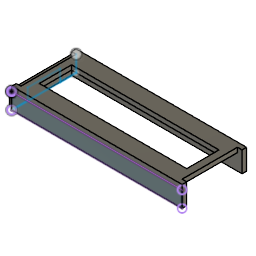
LCD Schutz (Autodesk Fusion 360 design; units mm, degrees)
part number: 2026-08-05-17-31-47-959
Autodesk Fusion 360 part; units mm, degrees
sketch "Sketch1" plane through (0, 0, 0) normal (0, 0, 1) x (1, 0, 0)
  line L0 (0, 0) -> (74, 0)
  line L1 (74, 0) -> (74, 28)
  line L2 (74, 28) -> (0, 28)
  line L3 (0, 28) -> (0, 0)
  line L4 (72, 26) -> (2, 26)
  line L5 (2, 26) -> (2, 2)
  line L6 (2, 2) -> (72, 2)
  line L7 (72, 2) -> (72, 26)
  line L8 (5, 7) -> (69, 7)
  line L9 (69, 7) -> (69, 21)
  line L10 (69, 21) -> (5, 21)
  line L11 (5, 21) -> (5, 7)
  dimension "d1" = 74
  dimension "d2" = 28
  dimension "d3" = 70
  dimension "d4" = 24
  dimension "d7" = 2
  dimension "d8" = 2
  dimension "d9" = 64
  dimension "d10" = 14
  dimension "d11" = 5
  dimension "d12" = 3
  constraint horizontal L0
  constraint vertical L1
  constraint horizontal L2
  constraint vertical L3
  constraint coincident L0.start L3.end
  constraint horizontal L4
  constraint vertical L5
  constraint horizontal L6
  constraint vertical L7
  constraint horizontal L8
  constraint vertical L9
  constraint horizontal L10
  constraint vertical L11
  measures "d1" distance of L0.start L0.end
  measures "d2" distance of L0.start L2.end
  measures "d3" distance of L4.start L4.end
  measures "d4" distance of L4.start L6.end
  measures "d7" distance of L2 L4
  measures "d8" distance of L1 L7
  measures "d9" distance of L8.start L8.end
  measures "d10" distance of L8.start L10.end
  measures "d11" distance of L4 L10
  measures "d12" distance of L5 L11
sketch "Sketch2" plane through (0, 0, 0) normal (0, 0, 1) x (1, 0, 0)
sketch "Sketch3" plane through (0, 0, 0) normal (0, 1, 0) x (1, 0, 0)
sketch "Sketch4" plane through (0, 0, 0) normal (0, 1, 0) x (1, 0, 0)
  line L0 (0, 0) -> (74, 0)
  line L1 (74, 0) -> (74, 7)
  line L2 (74, 7) -> (0, 7)
  line L3 (0, 7) -> (0, 0)
  dimension "d13" = 74
  dimension "d14" = 7
  constraint horizontal L0
  constraint vertical L1
  constraint horizontal L2
  constraint vertical L3
  constraint coincident L0.start L3.end
  measures "d13" distance of L0.start L0.end
  measures "d14" distance of L0.start L2.end
sketch "Sketch5" plane through (0, 0, 0) normal (1, 0, 0) x (0, 1, 0)
  line L0 (28, 0) -> (28, -7)
  line L1 (28, -7) -> (0, -7)
  line L2 (0, -7) -> (0, 0)
  constraint vertical L0
  constraint horizontal L1
  constraint vertical L2
  constraint coincident L2.end origin
sketch "Sketch6" plane through (0, 0, 0) normal (0, 1, 0) x (1, 0, 0)
  line L0 (0, 0) -> (74, 0)
  line L1 (74, 0) -> (74, 7)
  line L2 (74, 7) -> (0, 7)
  line L3 (0, 7) -> (0, 0)
  constraint horizontal L0
  constraint vertical L1
  constraint horizontal L2
  constraint vertical L3
  constraint coincident L0.start L3.end
sketch "Sketch7" plane through (0, 0, 0) normal (0, 1, 0) x (1, 0, 0)
  line L0 (0, 0, 28) -> (74, 0, 28)
  line L1 (74, 0, 28) -> (74, 7, 28)
  line L2 (74, 7, 28) -> (0, 7, 28)
  line L3 (0, 7, 28) -> (0, 0, 28)
  dimension "d15" = 74
sketch "Sketch8" plane through (0, 0, 0) normal (1, 0, 0) x (0, 1, 0)
  line L0 (0, -7) -> (7, -7)
  line L1 (7, -7) -> (7, -2)
  line L2 (7, -2) -> (21, -2)
  line L3 (21, -2) -> (21, -7)
  line L4 (21, -7) -> (28, -7)
  dimension "d16" = 7
  dimension "d17" = 5
  constraint horizontal L0
  constraint perpendicular L0 L1
  constraint perpendicular L1 L2
  constraint perpendicular L2 L3
  constraint perpendicular L1 L4
  measures "d16" distance of L0.start L0.end
  measures "d17" distance of L2.end L3.end
sketch "Sketch9" plane through (0, 28, 0) normal (0, 1, 0) x (1, 0, 0)
sketch "Sketch10" plane through (0, 0, 0) normal (1, 0, 0) x (0, 1, 0)
  line L0 (0, 0) -> (28, 0)
  line L1 (28, 0) -> (28, -7)
  line L2 (28, -7) -> (0, -7)
  line L3 (0, -7) -> (0, 0)
  constraint horizontal L0
  constraint vertical L1
  constraint horizontal L2
  constraint vertical L3
  constraint coincident L0.start L3.end
sketch "Sketch11" plane through (0, 0, 0) normal (0, 0, 1) x (1, 0, 0)
sketch "Sketch12" plane through (0, 0, 0) normal (1, 0, 0) x (0, 1, 0)
  line L0 (0, -7) -> (28, -7)
  line L1 (28, -7) -> (28, 0)
  constraint horizontal L0
  constraint perpendicular L0 L1
sketch "Sketch13" plane through (0, 0, 0) normal (0, 1, 0) x (1, 0, 0)
  line L0 (74, 7) -> (0, 7)
  line L1 (0, 0) -> (74, 0)
  dimension "d18" = 7
  measures "d18" distance of L0 L1
sketch "Sketch14" plane through (0, 0, 0) normal (0, 1, 0) x (1, 0, 0)
extrude "Extrude1" add sketch "Sketch6" along normal blind 2 makes body 1
extrude "Extrude2" add sketch "Sketch7" against normal blind 2 separate body contours L0 L1 L2 L3 in plane through (0, 28, 0) normal (0, 1, 0) makes body 2
extrude "Extrude3" add sketch "Sketch1" along normal blind 1 contours L4 L5 L6 L7 bodies 1 2
extrude "Extrude4" add 1 faces at (25.3333, 0.6667, 0) along direction (0, 0, 1) blind 1 on bodies 1 bodies 1
extrude "Extrude5" add 1 faces at (25.3333, 27.3333, 0) along direction (0, 0, 1) blind 1 on bodies 1 bodies 1
extrude "Extrude6" add sketch "Sketch10" against normal blind 1 bodies 1
sketch "Sketch15" plane through (0, 0, 0) normal (1, 0, 0) x (0, 1, 0)
sketch "Sketch16" plane through (0, 0, 0) normal (1, 0, 0) x (0, 1, 0)
extrude "Extrude7" add 1 faces at (47.6667, 3.6667, 1) along direction (0, 0, 1) blind 1 on bodies 1 bodies 1
